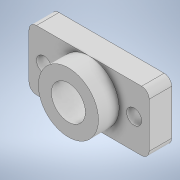
# Autodesk Inventor part: M5Nut_Special
Saved by Autodesk Inventor 2020.2 (Build 242310000, 310)
## iProperties
Created: 2019-09-01
Part Number: M5Nut_Special
Material: Generic
Document SubType Name: Modeling
Designer: victo
Density: 1 g/cm^3
Appearance: Default
Author: victo
Autodesk Inventor part; units mm, degrees
ref_plane "YZ Plane" through (0, 0, 0) normal (1, 0, 0) x (0, 1, 0)
ref_plane "XZ Plane" through (0, 0, 0) normal (0, 1, 0) x (-1, 0, 0)
ref_plane "XY Plane" through (0, 0, 0) normal (0, 0, 1) x (1, 0, 0)
sketch "Sketch1" plane through (0, 0, 0) normal (0, 0, 1) x (1, 0, 0)
  circle A0 centre (0, 0) radius 4
  circle A1 centre (0, 0) radius 2.26
  dimension "d0" = 8
  dimension "d1" = 4.52
  constraints: 2 centre point, 2 coincident
  measures "d0" diameter of A0
  measures "d1" diameter of A1
extrude "Extrusion1" add sketch "Sketch1" along normal blind 5.75
sketch "Sketch2" plane through (0, 0, 0) normal (0, 0, -1) x (-1, 0, 0)
  circle A0 centre (0, 0) radius 2.26 projected
  circle A1 centre (6, 0) radius 1
  circle A2 centre (-6, 0) radius 1
  line L0 (8, 4) -> (-8, 4)
  line L1 (-8, 4) -> (-8, -4)
  line L2 (-8, -4) -> (8, -4)
  line L3 (8, -4) -> (8, 4)
  line L4 (8, 4) -> (-8, -4) construction
  line L5 (-8, 4) -> (8, -4) construction
  dimension "d7" = 2
  dimension "d8" = 2
  dimension "d9" = 6
  dimension "d10" = 6
  dimension "d11" = 0
  dimension "d12" = 0
  dimension "d19" = 16
  dimension "d20" = 8
  constraints: 12 end point, 2 centre point, 2 midpoint, 2 parallel, 1 horizontal, 1 perpendicular
  measures "d7" diameter of A1
  measures "d8" diameter of A2
  measures "d9" distance of A1.centre point (0, 0)
  measures "d10" distance of point (0, 0) A2.centre
  measures "d11" vertical distance of A1.centre point (0, 0)
  measures "d12" vertical distance of point (0, 0) A2.centre
  measures "d19" distance of L2.end L1.end
  measures "d20" distance of L1.end L0.end
extrude "Extrusion2" add sketch "Sketch2" against normal blind 3
fillet "Fillet1" radius 1 4 edges at (8, 4, 1.5) (8, -4, 1.5) (-8, -4, 1.5) (-8, 4, 1.5)
equation "\"d29\" = 55deg"
equation "\"Sketch3_Pitch\" = 0.8"
equation "\"d47\" = 55deg"
equation "\"Sketch5_Pitch\" = 0.4"
equation "\"d65\" = 55deg"
equation "\"Sketch7_Pitch\" = 0.4"
body "Solid1"
